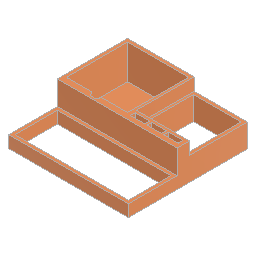
Writing-Equipment-Structure (Autodesk Fusion 360 design; units mm, degrees)
Autodesk Fusion 360 part; units mm, degrees
sketch "Sketch3" plane through (0, 0, 48.175) normal (0, 0, 1) x (-1, 0, 0)
  line L0 (-154.55, 230.942) -> (-136.55, 230.942)
  line L1 (-136.55, 230.942) -> (-136.55, 224.942)
  line L2 (-136.55, 224.942) -> (-154.55, 224.942)
  line L3 (-154.55, 224.942) -> (-154.55, 230.942)
  arc A0 (-131.55, 154.472) -> (-130.05, 152.972) centre (-130.05, 154.472) ccw
  line L4 (-131.55, 154.472) -> (-131.55, 227.922)
  arc A1 (-130.05, 229.422) -> (-131.55, 227.922) centre (-130.05, 227.922) ccw
  line L5 (-130.05, 229.422) -> (-100.725, 229.422)
  arc A2 (-100.725, 229.422) -> (-98.225, 231.922) centre (-100.725, 231.922) ccw
  arc A3 (-95.7304, 234.422) -> (-98.225, 231.922) centre (-95.7304, 231.9274) ccw
  line L6 (-95.7304, 234.422) -> (-90.7304, 234.422)
  arc A4 (-88.225, 231.922) -> (-90.7304, 234.422) centre (-90.7304, 231.9166) ccw
  arc A5 (-88.225, 231.922) -> (-85.725, 229.422) centre (-85.725, 231.922) ccw
  line L7 (-85.725, 229.422) -> (-56.6, 229.422)
  arc A6 (-55.1, 227.922) -> (-56.6, 229.422) centre (-56.6, 227.922) ccw
  line L8 (-55.1, 227.922) -> (-55.1, 152.972)
  line L9 (-55.1, 152.972) -> (-130.05, 152.972)
  line L10 (-157.4, 224.942) -> (-175.4, 224.942)
  line L11 (-175.4, 224.942) -> (-175.4, 230.942)
  line L12 (-175.4, 230.942) -> (-157.4, 230.942)
  line L13 (-157.4, 230.942) -> (-157.4, 224.942)
  line L14 (-178.25, 224.942) -> (-196.25, 224.942)
  line L15 (-196.25, 224.942) -> (-196.25, 230.942)
  line L16 (-196.25, 230.942) -> (-178.25, 230.942)
  line L17 (-178.25, 230.942) -> (-178.25, 224.942)
  line L18 (-163, 218.046) -> (-137.55, 218.046)
  line L19 (-137.55, 218.046) -> (-137.55, 152.972)
  line L20 (-137.55, 152.972) -> (-163, 152.972)
  line L21 (-163, 152.972) -> (-163, 218.046)
  line L22 (-171.65, 218.046) -> (-171.65, 152.972)
  line L23 (-171.65, 152.972) -> (-197.1, 152.972)
  line L24 (-197.1, 152.972) -> (-197.1, 218.046)
  line L25 (-197.1, 218.046) -> (-171.65, 218.046)
  line L26 (-51.1, 236.942) -> (-201.1, 236.942)
  line L27 (-201.1, 236.942) -> (-201.1, 148.972)
  line L28 (-201.1, 148.972) -> (-51.1, 148.972)
  line L29 (-51.1, 148.972) -> (-51.1, 236.942)
  line L30 (-201.1, 148.972) -> (-134.55, 148.972)
  line L31 (-134.55, 148.972) -> (-134.55, 221.472)
  line L32 (-134.55, 221.472) -> (-201.1, 221.472)
  line L33 (-201.1, 221.472) -> (-201.1, 148.972)
  point P0 (-201.1, 148.972)
  dimension "d1" = 66.55
  dimension "d2" = 72.5
  constraint horizontal L30
  constraint vertical L31
  constraint horizontal L32
  constraint vertical L33
  constraint coincident P0 L27.end
  measures "d1" distance of P0 L30.end
  measures "d2" distance of P0 L32.end
sketch "Sketch1" plane through (0, 0, 3.175) normal (0, 0, 1) x (-1, 0, 0)
  line L0 (0, 0) -> (0, 297.942)
  line L1 (0, 297.942) -> (-407.924, 297.942)
  line L2 (-407.924, 297.942) -> (-407.924, 0)
  line L3 (-407.924, 0) -> (0, 0)
  line L4 (-51.1, 297.942) -> (-51.1, 148.972)
  line L5 (-51.1, 148.972) -> (0, 148.972)
  line L6 (-51.1, 297.942) -> (-201.1, 297.942)
  line L7 (-201.1, 297.942) -> (-201.1, 148.972)
  line L8 (-201.1, 148.972) -> (-51.1, 148.972)
  line L9 (-51.1, 148.972) -> (-51.1, 297.942)
  line L10 (-55.1, 293.942) -> (-197.1, 293.942)
  line L11 (-55.1, 240.942) -> (-197.1, 240.942)
  line L12 (-55.1, 236.942) -> (-197.1, 236.942)
  line L13 (-55.1, 152.972) -> (-55.1, 227.922)
  line L14 (-55.1, 240.942) -> (-55.1, 293.942)
  line L15 (-197.1, 293.942) -> (-197.1, 240.942)
  line L16 (-197.1, 236.942) -> (-201.1, 236.942)
  line L17 (-55.1, 236.942) -> (-51.1, 236.942)
  line L18 (-55.1, 152.972) -> (-130.05, 152.972)
  line L19 (-131.55, 154.472) -> (-131.55, 227.922)
  line L20 (-55.1, 229.422) -> (-55.1, 154.472)
  line L21 (-130.05, 229.422) -> (-100.725, 229.422)
  line L22 (-85.725, 229.422) -> (-56.6, 229.422)
  line L23 (-95.7304, 234.422) -> (-90.7304, 234.422)
  arc A0 (-100.725, 229.422) -> (-98.225, 231.922) centre (-100.725, 231.922) ccw
  arc A1 (-95.7304, 234.422) -> (-98.225, 231.922) centre (-95.7304, 231.9274) ccw
  arc A2 (-88.225, 231.922) -> (-90.7304, 234.422) centre (-90.7304, 231.9166) ccw
  arc A3 (-88.225, 231.922) -> (-85.725, 229.422) centre (-85.725, 231.922) ccw
  arc A4 (-130.05, 229.422) -> (-131.55, 227.922) centre (-130.05, 227.922) ccw
  arc A5 (-131.55, 154.472) -> (-130.05, 152.972) centre (-130.05, 154.472) ccw
  arc A6 (-56.6, 152.972) -> (-55.1, 154.472) centre (-56.6, 154.472) ccw
  arc A7 (-55.1, 227.922) -> (-56.6, 229.422) centre (-56.6, 227.922) ccw
  line L24 (-55.1, 234.942) -> (-55.1, 227.922)
  line L25 (-130.05, 152.972) -> (-56.6, 152.972)
  line L26 (-137.55, 152.972) -> (-163, 152.972)
  line L27 (-163, 152.972) -> (-163, 218.046)
  line L28 (-163, 218.046) -> (-137.55, 218.046)
  line L29 (-137.55, 218.046) -> (-137.55, 152.972)
  line L30 (-197.1, 152.972) -> (-197.1, 218.046)
  line L31 (-197.1, 218.046) -> (-171.65, 218.046)
  line L32 (-171.65, 218.046) -> (-171.65, 152.972)
  line L33 (-171.65, 152.972) -> (-197.1, 152.972)
  line L34 (-136.55, 224.942) -> (-154.55, 224.942)
  line L35 (-154.55, 224.942) -> (-154.55, 230.942)
  line L36 (-154.55, 230.942) -> (-136.55, 230.942)
  line L37 (-136.55, 230.942) -> (-136.55, 224.942)
  line L38 (-157.4, 224.942) -> (-175.4, 224.942)
  line L39 (-157.4, 230.942) -> (-157.4, 224.942)
  line L40 (-175.4, 230.942) -> (-157.4, 230.942)
  line L41 (-175.4, 224.942) -> (-175.4, 230.942)
  line L42 (-178.25, 224.942) -> (-196.25, 224.942)
  line L43 (-178.25, 230.942) -> (-178.25, 224.942)
  line L44 (-196.25, 230.942) -> (-178.25, 230.942)
  line L45 (-196.25, 224.942) -> (-196.25, 230.942)
  point P0 (-131.55, 152.972)
  point P1 (-93.225, 229.422)
  point P2 (-98.225, 231.922)
  point P3 (-88.225, 231.922)
  point P4 (-90.7304, 234.422)
  point P5 (-95.7304, 234.422)
  dimension "d20" = 148.97
  dimension "d21" = 150
  dimension "d27" = 53
  dimension "d32" = 76.45
  dimension "d33" = 76.45
  dimension "d34" = 7.5
  dimension "d35" = 7.5
  dimension "d41" = 2.5
  dimension "d42" = 2.5
  dimension "d43" = 2.5
  dimension "d44" = 2.5
  dimension "d45" = 5
  dimension "d46" = 5
  dimension "d47" = 1.5
  dimension "d48" = 1.5
  dimension "d49" = 1.5
  dimension "d50" = 1.5
  dimension "d62" = 25.45
  dimension "d63" = 65.074
  dimension "d64" = 4
  dimension "d65" = 6
  dimension "d68" = -34.1
  dimension "d69" = 0
  dimension "d71" = 4
  dimension "d72" = 18
  dimension "d73" = 6
  dimension "d75" = 5
  dimension "d76" = 6
  dimension "d79" = -20.85
  dimension "d80" = 0
  constraint horizontal L6
  constraint vertical L7
  constraint horizontal L8
  constraint vertical L9
  constraint coincident L4.start L6.start
  constraint coincident L11.start L13
  constraint perpendicular L11 L15
  constraint collinear L13 L14
  constraint coincident L7 L16.end
  constraint perpendicular L7 L16
  constraint coincident L9 L17.end
  constraint perpendicular L9 L17
  constraint horizontal L18
  constraint vertical L19
  constraint horizontal L21
  constraint vertical L20
  constraint coincident L13 L18.start
  constraint coincident L22.start L21
  constraint collinear L21 L22
  constraint coincident P1 L21
  constraint coincident P5 L23.start
  constraint coincident P4 L23.end
  constraint tangent L21 A0
  constraint coincident P2 A0.end
  constraint tangent L23 A1
  constraint tangent L23 A2
  constraint coincident P3 A2.start
  constraint tangent L22 A3
  constraint tangent L21 A4
  constraint tangent L19 A4
  constraint coincident P0 L19
  constraint coincident P0 L18
  constraint tangent L19 A5
  constraint tangent L18 A5
  constraint coincident L13.start L20
  constraint tangent L20 A6
  constraint coincident L20.start L22
  constraint coincident L13 L24.start
  constraint tangent L22 A7
  constraint tangent L13 A7
  constraint horizontal L26
  constraint vertical L27
  constraint horizontal L28
  constraint vertical L29
  constraint horizontal L34
  constraint vertical L35
  constraint horizontal L36
  constraint vertical L37
  measures "d20" distance of L6.end L7.end
  measures "d21" distance of L4.start L6.end
  measures "d27" distance of L10 L11
  measures "d32" distance of L13.start P0
  measures "d33" distance of L13.start L20.start
  measures "d34" distance of P1 L21.end
  measures "d35" distance of P1 L22.start
  measures "d41" horizontal distance of L21.end P2
  measures "d42" distance of P2 L21
  measures "d43" distance of P3 L21
  measures "d44" horizontal distance of L22.start P3
  measures "d45" distance of L21 P5
  measures "d46" distance of L22 P4
  measures "d47" radius of A4
  measures "d48" radius of A5
  measures "d49" radius of A6
  measures "d50" radius of A7
  measures "d62" distance of L26.start L26.end
  measures "d63" distance of L26.start L28.end
  measures "d64" distance of L8 L26
  measures "d65" distance of L19 L29
  measures "d71" distance of L7 L30
  measures "d72" distance of L34.start L34.end
  measures "d73" distance of L34.start L36.end
  measures "d75" distance of L19 L37
  measures "d76" distance of L12 L36
extrude "Extrude1" add sketch "Sketch1" along normal blind 15 contours L1 L4 L6 L7 L9 L12 L16 L17
extrude "Extrude2" add sketch "Sketch1" along normal blind 45 contours L4 L7 L8 L9 L12 L16 L17
extrude "Extrude3" add sketch "Sketch1" along normal blind 2 contours L13 L18 L19 L20 L21 L22 L23 A0 A1 A2 A3 A4 A5 A6 A7 L25
extrude "Extrude4" cut sketch "Sketch3" against normal blind 15.7 contours L27 L28 L30 L31 L32 L33
sketch "Sketch2" plane through (0, 0, 32.475) normal (0, 0, 1) x (-1, 0, 0)
  line L0 (-197.1, 152.972) -> (-197.1, 218.046)
  line L1 (-197.1, 218.046) -> (-171.65, 218.046)
  line L2 (-171.65, 218.046) -> (-171.65, 152.972)
  line L3 (-171.65, 152.972) -> (-197.1, 152.972)
  line L4 (-137.55, 152.972) -> (-163, 152.972)
  line L5 (-163, 152.972) -> (-163, 218.046)
  line L6 (-163, 218.046) -> (-137.55, 218.046)
  line L7 (-137.55, 218.046) -> (-137.55, 152.972)
  line L8 (-201.1, 221.472) -> (-201.1, 148.972)
  line L9 (-201.1, 148.972) -> (-134.55, 148.972)
  line L10 (-134.55, 148.972) -> (-134.55, 221.472)
  line L11 (-134.55, 221.472) -> (-201.1, 221.472)
  line L12 (-171.65, 218.046) -> (-163, 218.046)
  line L13 (-163, 152.972) -> (-171.65, 152.972)
  constraint coincident L1.end L2.start
  constraint coincident L5.end L6.start
  constraint coincident L4.end L5.start
  constraint coincident L2.end L3.start
extrude "Extrude5" cut sketch "Sketch2" against normal up to surface (29.3 mm away) contours L2 L5 L12 L13
equation "d20 = WritingEquipmentLength"
equation "d21 = WritingEquipmentWidth"
equation "d27 = PenLength"
equation "d28 = -ComponentWallWidth"
equation "d32 = PostItSquare + SmallTolerence * 4"
equation "d33 = PostItSquare + SmallTolerence * 4"
equation "d62 = EraserWidth"
equation "d63 = EraserLength"
equation "d64 = ComponentWallWidth"
equation "d65 = ComponentWallWidth * 1.5"
equation "d68 = -EraserWidth - 8.65 mm"
equation "d72 = PencilLeadLength"
equation "d73 = PencilLeadWidth"
equation "d79 = -PencilLeadLength - 2.85 mm"
equation "d90 = -EraserDepth - 3 mm"
equation "ComponentWallWidth = 4 mm"
equation "WritingEquipmentLength = 148.97 mm"
equation "WritingEquipmentWidth = 150 mm"
equation "PenLength = 53 mm"
equation "SmallTolerence = 0.05 mm"
equation "PostItSquare = 76.2 mm + SmallTolerence"
equation "PencilLeadWidth = 6 mm"
equation "PencilLeadLength = 18 mm"
equation "EraserLength = 2.56 in + SmallTolerence"
equation "EraserWidth = 1 in + SmallTolerence"
equation "EraserDepth = 0.5 in"
equation "d1 = 63.550 mm + 3 mm"
equation "d2 = 69 mm + 3.5 mm"
